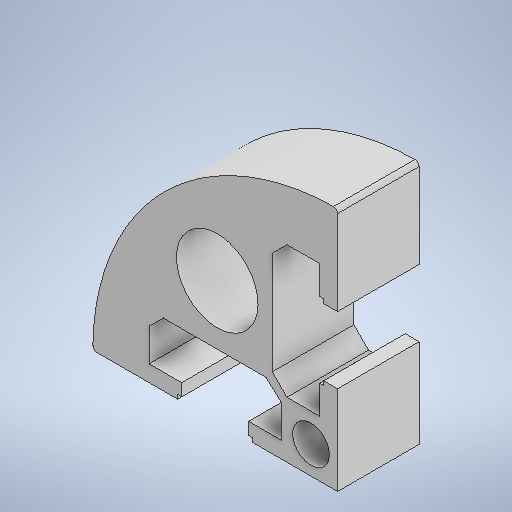
# Autodesk Inventor part: profile_30x30_R90
Saved by Autodesk Inventor 2025.2 (Build 292293000, 293)
## iProperties
Created: 2025-04-07
Part Number: profile_30x30_R90
Material: Generic
Document SubType Name: Modeling
Designer: kenne
Density: 1 g/cm^3
Appearance: Default
Author: kenne
Autodesk Inventor part; units mm, degrees
ref_plane "YZ Plane" through (0, 0, 0) normal (1, 0, 0) x (0, 1, 0)
ref_plane "XZ Plane" through (0, 0, 0) normal (0, 1, 0) x (-1, 0, 0)
ref_plane "XY Plane" through (0, 0, 0) normal (0, 0, 1) x (1, 0, 0)
sketch "Sketch1" plane through (0, 0, 0) normal (0, 0, 1) x (1, 0, 0)
  line L0 (-14.7479, -15) -> (14.7479, -15) construction
  circle A0 centre (0, 0) radius 5
  line L1 (14.7479, 0) -> (14.7479, 4.1) construction
  line L2 (12.5479, 4.1) -> (14.7479, 4.1) construction
  line L3 (28.5, 15) -> (28.5, -15) construction
  line L4 (14.7479, 14.4958) -> (14.7479, 4.1)
  line L5 (6.7479, 15) -> (14.7479, 15) construction
  line L6 (12.5479, 8.1) -> (12.5479, 4.1) construction
  line L7 (8.5479, 8.1) -> (12.5479, 8.1)
  line L8 (6.7479, 15) -> (6.7479, -13) construction
  line L9 (8.5479, 8.1) -> (6.7479, 6.3)
  line L10 (6.7479, 6.3) -> (6.7479, 0)
  line L11 (6.7479, 0) -> (6.7479, -6.3)
  line L12 (6.7479, -6.3) -> (8.5479, -8.1)
  line L13 (8.5479, -8.1) -> (12.5479, -8.1)
  line L14 (12.5479, -4.1) -> (12.5479, -8.1) construction
  line L15 (12.5479, -4.1) -> (14.7479, -4.1) construction
  line L16 (14.7479, -4.1) -> (14.7479, -15)
  circle A1 centre (11.5, -11.6) radius 2.25
  line L17 (14.7479, -15) -> (3.8479, -15) construction
  line L18 (3.8479, -15) -> (3.8479, -13) construction
  line L19 (3.8479, -13) -> (7.8479, -13)
  line L20 (7.8479, -13) -> (7.8479, -9)
  line L21 (5.9801, -7.2704) -> (7.8479, -9)
  arc A2 (14.2394, 14.9957) -> (-15.2478, -14.4915) centre (14.7479, -15) ccw
  line L22 (-15.2521, -15) -> (-4.3521, -15) construction
  line L23 (-4.3521, -15) -> (-4.3521, -13) construction
  line L24 (-4.3521, -13) -> (-8.3521, -13)
  line L25 (-8.3521, -13) -> (-8.3521, -9)
  line L26 (-6.6199, -7.2704) -> (5.9801, -7.2704)
  line L27 (-8.3521, -9) -> (-6.6199, -7.2704)
  line L28 (-4.3521, -15) -> (-4.8521, -15) construction
  line L29 (-4.8521, -15) -> (-4.8521, -14.5)
  line L30 (-4.8521, -14.5) -> (-4.3521, -14.5)
  line L31 (-4.3521, -14.5) -> (-4.3521, -15) construction
  line L32 (-4.3521, -14.5) -> (-4.3521, -13)
  line L33 (-4.8521, -15) -> (-15.2521, -15)
  line L34 (12.5479, 4.1) -> (13.0479, 4.1) construction
  line L35 (13.0479, 4.1) -> (13.0479, 4.6)
  line L36 (13.0479, 4.6) -> (12.5479, 4.6)
  line L37 (12.5479, 4.6) -> (12.5479, 4.1) construction
  line L38 (12.5479, 8.1) -> (12.5479, 4.6)
  line L39 (13.0479, 4.1) -> (14.7479, 4.1)
  line L40 (12.5479, -4.1) -> (13.0479, -4.1) construction
  line L41 (13.0479, -4.1) -> (13.0479, -4.6)
  line L42 (13.0479, -4.6) -> (12.5479, -4.6)
  line L43 (12.5479, -4.6) -> (12.5479, -4.1) construction
  line L44 (14.7479, -4.1) -> (13.0479, -4.1)
  line L45 (12.5479, -8.1) -> (12.5479, -4.6)
  line L46 (3.8479, -15) -> (4.3479, -15) construction
  line L47 (4.3479, -15) -> (4.3479, -14.5)
  line L48 (4.3479, -14.5) -> (3.8479, -14.5)
  line L49 (3.8479, -14.5) -> (3.8479, -15) construction
  line L50 (3.8479, -13) -> (3.8479, -14.5)
  line L51 (14.7479, -15) -> (4.3479, -15)
  circle A3 centre (0, 0) radius 7 construction
  line L52 (-7.9343, -5.7565) -> (-9.5924, -7.4121)
  line L53 (-6.5211, -5.1718) -> (-5.3487, -5.1718) construction
  line L54 (-5.3487, -5.1718) -> (-5.3487, -4.5157) construction
  line L55 (-10.1792, -8.8274) -> (-10.1792, -13)
  arc A4 (-6.655, 2.1705) -> (-5.3487, -4.5157) centre (0, 0) ccw construction
  line L56 (-10.6792, -13.5) -> (-13.2083, -13.5)
  arc A5 (-9.5924, -7.4121) -> (-10.1792, -8.8274) centre (-8.1792, -8.8274) ccw
  arc A6 (-6.5211, -5.1718) -> (-7.9343, -5.7565) centre (-6.5211, -7.1718) ccw
  arc A7 (-6.655, 2.1705) -> (-13.7077, -13.0232) centre (4.3732, -12.1825) ccw construction
  arc A8 (-6.9939, 0.2917) -> (-8.2035, 0.835) centre (-7.7074, 0.3214) ccw
  arc A9 (-6.9939, 0.2917) -> (-5.3487, -4.5157) centre (0, 0) ccw construction
  arc A10 (-8.2035, 0.835) -> (-13.6792, -13.5) centre (4.3732, -12.1825) ccw
  arc A11 (-13.7077, -13.0232) -> (-13.2083, -13.5) centre (-13.2083, -13) ccw
  arc A12 (-10.6792, -13.5) -> (-10.1792, -13) centre (-10.6792, -13) ccw
  arc A13 (-15.2478, -14.4915) -> (-14.7479, -15) centre (-14.7479, -14.5) ccw
  arc A14 (14.7479, 14.4958) -> (14.2394, 14.9957) centre (14.2479, 14.4958) ccw
  arc A15 (-5.3487, -4.8273) -> (-5.5333, -4.2875) centre (-6.23, -4.8273) ccw construction
  arc A16 (-5.5751, -5.1718) -> (-5.3487, -4.9454) centre (-5.5751, -4.9454) ccw construction
  arc A17 (-6.9939, 0.2917) -> (-5.5333, -4.2875) centre (0, 0) ccw
  arc A18 (-5.3487, -4.8273) -> (-5.5333, -4.2875) centre (-6.23, -4.8273) ccw
  arc A19 (-5.5751, -5.1718) -> (-5.3487, -4.9454) centre (-5.5751, -4.9454) ccw
  line L57 (-5.3487, -4.8273) -> (-5.3487, -4.9454)
  line L58 (-5.5751, -5.1718) -> (-6.5211, -5.1718)
  point P0 (0, -15)
  point P1 (28.5, 0)
  point P2 (14.7479, -15)
  point P3 (-10.1792, -7.9981)
  point P4 (-7.3487, -5.1718)
  point P5 (-10.1792, -13.5)
  point P6 (-9.8021, -15)
  point P7 (-14.7479, -15)
  dimension "d0" = 30
  dimension "d2" = 10
  dimension "d3" = 4.1
  dimension "d4" = 2.2
  dimension "d5" = 30
  dimension "d6" = 28.5
  dimension "d7" = 8
  dimension "d8" = 4
  dimension "d9" = 28
  dimension "d10" = 45
  dimension "inner_width" = 6.3
  dimension "d12" = 6.3
  dimension "d13" = 45
  dimension "d15" = 4.5
  dimension "d16" = 11.5
  dimension "d17" = 3.5
  dimension "d18" = 2
  dimension "d19" = 4
  dimension "d20" = 4
  dimension "d21" = 2.2
  dimension "d22" = 30
  dimension "d23" = 10.9
  dimension "d24" = 12.6
  dimension "d25" = 0.5
  dimension "d26" = 0.5
  dimension "d27" = 0.5
  dimension "d28" = 0.5
  dimension "d31" = 2
  dimension "d32" = 4
  dimension "d33" = 2
  dimension "d34" = 2
  dimension "d35" = 0.6561
  dimension "d36" = 1.5
  dimension "d37" = 2
  dimension "d38" = 3.5
  dimension "d39" = 18.1005
  dimension "d40" = 2.8175
  dimension "d41" = 0.7141
  dimension "d42" = 0.5
  dimension "d43" = 0.8813
  dimension "d44" = 0.2265
  constraints: 119 end point, 42 point on circle, 20 centre point, 19 tangent, 16 point on line, 15 horizontal, 14 equal length, 13 vertical, 9 equal radius, 9 parallel, 9 perpendicular, 4 collinear, 4 horizontal alignment, 3 midpoint, 2 coincident, 2 vertical alignment
  measures "d0" distance of L22.start L0.end
  measures "d2" diameter of A0
  measures "d3" distance of L1.start L1.end
  measures "d4" distance of L2.start L1.end
  measures "d5" distance of L3.start L3.end
  measures "d6" distance from line of L3 point (0, 0)
  measures "d7" distance of L5.start L5.end
  measures "d8" distance of L6.start L2.start
  measures "d9" distance of L5.start L8.end
  measures "d10" angle of L8 L9
  measures "inner_width" distance of L9.end L10.end
  measures "d12" distance of L10.end L11.end
  measures "d13" angle of L8 L12
  measures "d15" diameter of A1
  measures "d16" horizontal distance of point (0, 0) A1.centre
  measures "d17" distance from line of A1.centre L13
  measures "d18" distance of L17.end L18.end
  measures "d19" distance of L18.end L19.end
  measures "d20" distance of L19.end L20.end
  measures "d21" angle of L21 L12
  measures "d22" radius of A2
  measures "d23" distance of L22.start L22.end
  measures "d24" distance of L21.start L26.start
  measures "d25" distance of L28.end L29.end
  measures "d26" distance of L36.end L35.end
  measures "d27" distance of L41.end L42.end
  measures "d28" distance of L48.end L47.end
  measures "d31" radial gap between concentric circles of A3 A0
  measures "d32" distance of point (-7.349, -5.172) point (-10.179, -7.998)
  measures "d33" distance between parallel lines of L27 L52
  measures "d34" distance of point (-7.349, -5.172) L53.end
  measures "d35" distance of L53.end L54.end
  measures "d36" vertical distance of point (-9.802, -15) point (-10.179, -13.5)
  measures "d37" radius of A5
  measures "d38" distance of point (-10.179, -13.5) A10.end
  measures "d39" radius of A7
  measures "d40" vertical distance of point (0, -15) A7.centre
  measures "d41" radius of A8
  measures "d42" radius of A11
  measures "d43" radius of A18
  measures "d44" radius of A16
extrude "Extrusion1" add sketch "Sketch1" along normal mid plane 10 contours L4 L39 L35 L36 L38 L7 L9 L10 L11 L12 L13 L45 L42 L41 L44 L16 L51 L47 L48 L50 L19 L20 L21 L26 L27 L25 L24 L32 L30 L29 L33 A13 A2 A14 | L52 A5 L55 A12 L56 A11 A10 A8 A17 A18 L57 A19 L58 A6
equation "\"d12\" = inner_width"
body "Solid1"
